Autodesk Fusion 360 part; units mm, degrees
note: some values were not read from the file. Set by a fixed rule: which face or edge a step refers to.
(part 3 of 4)
  circle A0 centre (-1.215, 0) radius 21.6
  circle A1 centre (-36.643, 0) radius 6.215
  circle A2 centre (-18.929, -30.6815) radius 6.215
  circle A3 centre (16.499, -30.6815) radius 6.215
  circle A4 centre (34.213, 0) radius 6.215
  circle A5 centre (16.499, 30.6815) radius 6.215
  circle A6 centre (-18.929, 30.6815) radius 6.215
  circle A7 centre (54, 0) radius 2
  circle A8 centre (53.3352, 8.4475) radius 2
  circle A9 centre (51.3571, 16.6869) radius 2
  circle A10 centre (48.1144, 24.5155) radius 2
  circle A11 centre (43.6869, 31.7404) radius 2
  circle A12 centre (38.1838, 38.1838) radius 2
  circle A13 centre (31.7404, 43.6869) radius 2
  circle A14 centre (24.5155, 48.1144) radius 2
  circle A15 centre (16.6869, 51.3571) radius 2
  circle A16 centre (8.4475, 53.3352) radius 2
  circle A17 centre (0, 54) radius 2
  circle A18 centre (-8.4475, 53.3352) radius 2
  circle A19 centre (-16.6869, 51.3571) radius 2
  circle A20 centre (-24.5155, 48.1144) radius 2
  circle A21 centre (-31.7404, 43.6869) radius 2
  circle A22 centre (-38.1838, 38.1838) radius 2
  circle A23 centre (-43.6869, 31.7404) radius 2
  circle A24 centre (-48.1144, 24.5155) radius 2
  circle A25 centre (-51.3571, 16.6869) radius 2
  circle A26 centre (-53.3352, 8.4475) radius 2
  circle A27 centre (-54, 0) radius 2
  circle A28 centre (-53.3352, -8.4475) radius 2
  circle A29 centre (-51.3571, -16.6869) radius 2
  circle A30 centre (-48.1144, -24.5155) radius 2
  circle A31 centre (-43.6869, -31.7404) radius 2
  circle A32 centre (-38.1838, -38.1838) radius 2
  circle A33 centre (-31.7404, -43.6869) radius 2
  circle A34 centre (-24.5155, -48.1144) radius 2
  circle A35 centre (-16.6869, -51.3571) radius 2
  circle A36 centre (-8.4475, -53.3352) radius 2
  circle A37 centre (0, -54) radius 2
  circle A38 centre (8.4475, -53.3352) radius 2
  circle A39 centre (16.6869, -51.3571) radius 2
  circle A40 centre (24.5155, -48.1144) radius 2
  circle A41 centre (31.7404, -43.6869) radius 2
  circle A42 centre (38.1838, -38.1838) radius 2
  circle A43 centre (43.6869, -31.7404) radius 2
  circle A44 centre (48.1144, -24.5155) radius 2
  circle A45 centre (51.3571, -16.6869) radius 2
  circle A46 centre (53.3352, -8.4475) radius 2
  circle A47 centre (-35.428, 0) radius 5
  circle A48 centre (-17.714, -30.6815) radius 5
  circle A49 centre (17.714, -30.6815) radius 5
  circle A50 centre (35.428, 0) radius 5
  circle A51 centre (17.714, 30.6815) radius 5
  circle A52 centre (-17.714, 30.6815) radius 5
  dimension "d277" = 35.428
  measures "d277" distance of origin A50.centre
sketch "outer teeth" plane through (0, 0, 0) normal (0, 0, 1) x (1, 0, 0) in component "ACG - Trapezoidal Profiles"
  line L0 (50.4, 0.75) -> (50.4, 0)
  circle A0 centre (0, 0) radius 55
  line L1 (54.9231, 2.9074) -> (50.4, 0.75)
  line L2 (0, 0) -> (55, 0) construction
  circle A1 centre (0, 0) radius 60
  line L3 (50.4, -0.75) -> (54.9231, -2.9074)
  line L4 (50.4, 0) -> (50.4, -0.75)
  dimension "d253" = 110
  dimension "d254" = 1.5
  dimension "d255" = 25.5
  dimension "d256" = 4.6
  dimension "d257" = 25.5
  dimension "d258" = 120
  constraint coincident A0.centre L2.start
  constraint coincident L2.end A0
  constraint horizontal L2
  constraint coincident L1.start A0
  constraint coincident L0.end L2
  constraint coincident L3.end A0
  constraint vertical L0
  constraint vertical L4
  constraint equal L0 L4
  measures "d253" diameter of A0
  measures "d254" distance of L3.start L0.start
  measures "d255" angle of L1 L2
  measures "d256" distance of L2.end L0
  measures "d257" angle of L2 L3
  measures "d258" diameter of A1
sketch "inner teeth" plane through (0, 0, 0) normal (0, 0, 1) x (1, 0, 0) in component "ACG - Trapezoidal Profiles"
  line L0 (2.7, 0) -> (50.046, 3.8222) construction
  line L1 (54.6914, 3.4447) -> (50.18, 1.3778)
  line L2 (2.7, 0) -> (50.2, 0) construction
  circle A0 centre (2.7, 0) radius 47.5
  line L3 (54.5707, 4.9399) -> (54.6914, 3.4447)
  line L4 (49.7862, 6.2564) -> (54.5707, 4.9399)
  point P0 (54.6311, 4.1923)
  dimension "d246" = 95
  dimension "d247" = 1.5
  dimension "d248" = 20
  dimension "d249" = 20
  dimension "d250" = 4.6
  dimension "d251" = 2.7
  dimension "d252" = 4.615
  constraint coincident L0.end A0
  constraint coincident L4.start A0
  constraint coincident L1.end A0
  constraint midpoint P0 L3
  constraint coincident L0.start L2.start
  constraint horizontal L0.start origin
  constraint coincident P0 L0
  constraint perpendicular L0 L3
  constraint coincident L2.end A0
  constraint horizontal L2
  measures "d246" diameter of A0
  measures "d247" distance of L1.start L3.start
  measures "d248" angle of L0 L4
  measures "d249" angle of L0 L1
  measures "d250" distance of L0.end L3
  measures "d251" distance of L0.start origin
  measures "d252" angle of L0 L2
sketch "Pins & Casing" plane through (0, 0, 0) normal (0, 0, 1) x (1, 0, 0) in component "Casing"
  circle A0 centre (-54, 0) radius 2
  circle A1 centre (0, 0) radius 55
  circle A2 centre (0, 0) radius 60
  line L0 (-35, -71) -> (-38.501, -76)
  line L1 (-60, -76) -> (-46.499, -76)
  line L2 (-60, -62) -> (-25, -42)
  circle A3 centre (0, 0) radius 15
  line L3 (-50, -71) -> (-35, -71)
  line L4 (-46.499, -76) -> (-50, -71)
  line L5 (50, -71) -> (46.499, -76)
  line L6 (-60, -80) -> (60, -80)
  line L7 (-60, -62) -> (60, -62)
  circle A4 centre (0, 0) radius 10
  line L8 (35, -71) -> (50, -71)
  line L9 (-38.501, -76) -> (38.501, -76)
  line L10 (46.499, -76) -> (60, -76)
  line L11 (25, -42) -> (60, -62)
  line L12 (-14.622, 3.3464) -> (-25, -42)
  line L13 (14.622, 3.3464) -> (25, -42)
  line L14 (38.501, -76) -> (35, -71)
  line L15 (-60, 0) -> (-60, -80)
  line L16 (60, -80) -> (60, 0)
  line L17 (54.9231, 2.9074) -> (50.4, 0.75)
  line L18 (50.4, 0.75) -> (50.4, 0)
  line L19 (50.4, 0) -> (50.4, -0.75)
  line L20 (50.4, -0.75) -> (54.9231, -2.9074)
  dimension "d9" = 110
  dimension "d10" = 120
  dimension "d33" = 80
  dimension "d34" = 30
  dimension "d35" = 20
  dimension "d36" = 55
  dimension "d37" = 55
  dimension "d38" = 55
  dimension "d39" = 55
  dimension "d40" = 4
  dimension "d41" = 5
  dimension "d42" = 10
  dimension "d43" = 15
  dimension "d44" = 18
  dimension "d45" = 20
  dimension "d50" = 25
  constraint coincident A1.centre A2.centre
  constraint perpendicular L6 L15
  constraint vertical L16
  constraint horizontal L6
  constraint coincident L2.start L15
  constraint coincident L7.end L16
  constraint coincident L13.start A3
  constraint coincident L12.start A3
  constraint tangent A3 L13
  constraint tangent A3 L12
  constraint coincident L1.start L15
  constraint perpendicular L1 L15
  constraint coincident L10.end L16
  constraint perpendicular L10 L16
  constraint horizontal L9
  constraint horizontal L3
  constraint horizontal L8
  constraint collinear L1 L9
  constraint collinear L9 L10
  constraint collinear L3 L8
  constraint equal L3 L8
  constraint equal L1 L10
  constraint horizontal L2.start L7.end
  constraint horizontal L2.end L11.start
  constraint equal L2 L11
  constraint coincident A2 L16.end
  constraint coincident A2 L15.start
  constraint tangent A2 L15
  constraint tangent A2 L16
  measures "d9" diameter of A1
  measures "d10" diameter of A2
  measures "d33" distance of A1.centre L6
  measures "d34" diameter of A3
  measures "d35" diameter of A4
  measures "d36" angle of L1 L4
  measures "d37" angle of L0 L9
  measures "d38" angle of L9 L14
  measures "d39" angle of L5 L10
  measures "d40" distance of L1 L6
  measures "d41" distance of L1 L3
  measures "d42" distance of L3.start L15
  measures "d43" distance of L3.start L0.start
  measures "d44" distance of L2.start L6
  measures "d45" vertical distance of L2.start L2.end
  measures "d50" horizontal distance of L2.end A1.centre
extrude "Extrude1" add sketch "Pins & Casing" against normal blind 5 contours A0 A1 | A0 A1 A2 L2 L11 | A1 L2 A3 L11 L12 L13 | A1 A2 L2 L11 | A2 L2 L15 | A2 L2 L7 L11 | A2 L11 L16 | L0 L1 L3 L4 L5 L7 L8 L9 L10 L14 L15 L16 | A3 | L0 L1 L3 L4 L5 L6 L8 L9 L10 L14 L15 L16 picked at (-55.3296, 0.0472) makes body 1 in component "Casing"
extrude "Extrude2" add sketch "Pins & Casing" against normal up to surface (5 mm away) contours A1 L17 L18 L19 L20 bodies 1 in component "Casing"
pattern_circular "C-Pattern1" count 40 over 360 about axis through (0, 0, 1.75) along (0, 0, 1) of "Extrude2" in component "Casing"
extrude "Extrude3" add sketch "Pins & Casing" along normal blind 24 contours A0 A1 | A0 A1 A2 L2 L11 | A1 A2 L2 L11 | A2 L2 L15 | A2 L2 L7 L11 | A2 L11 L16 | L0 L1 L3 L4 L5 L7 L8 L9 L10 L14 L15 L16 | L0 L1 L3 L4 L5 L6 L8 L9 L10 L14 L15 L16 picked at (-55.3296, 0.0472) bodies 1 in component "Casing"
extrude "Extrude7" add sketch "Pins & Casing" along normal up to surface (24 mm away) contours A1 L17 L18 L19 L20 bodies 1 in component "Casing"
fillet "Fillet3" radius 1 2 edges at (50.4, 0.75, 9.5) (50.4, -0.75, 9.5) on bodies 1 in component "Casing"
fillet "Fillet4" radius 1 2 edges at (54.9231, 2.9074, 9.5) (54.9231, -2.9074, 9.5) on bodies 1 in component "Casing"
pattern_circular "C-Pattern2" count 40 over 360 about axis through (0, 0, 1.75) along (0, 0, 1) of "Extrude7", "Fillet3", "Fillet4" in component "Casing"
extrude "Extrude8" add sketch "Pins & Casing" along normal blind 25 from surface at 24 contours L0 L1 L3 L4 L5 L7 L8 L9 L10 L14 L15 L16 | L0 L1 L3 L4 L5 L6 L8 L9 L10 L14 L15 L16 bodies 1 in component "Casing"
extrude "Extrude4" cut sketch "Pins & Casing" against normal blind 30 from surface at 49 contours L0 L1 L3 L4 L5 L6 L8 L9 L10 L14 L15 L16 bodies 1 in component "Casing"
extrude "Extrude5" add sketch "Pins & Casing" along normal up to surface (30 mm away) from surface at 19 separate body contours L0 L1 L3 L4 L5 L6 L8 L9 L10 L14 L15 L16 makes body 2 in component "Casing"
extrude "Extrude6" add sketch "Pins & Casing" along normal blind 5 from surface at 49 contours A1 L2 A3 L11 L12 L13 | A1 A2 L2 L11 | A2 L2 L7 L11 | L0 L1 L3 L4 L5 L7 L8 L9 L10 L14 L15 L16 | A3 | L0 L1 L3 L4 L5 L6 L8 L9 L10 L14 L15 L16 bodies 2 in component "Casing"
fillet "Fillet1" radius 0.6 4 edges at (50, -71, 34) (35, -71, 34) (-35, -71, 34) (-50, -71, 34) on bodies 2 in component "Casing"
fillet "Fillet2" radius 0.6 4 edges at (-46.499, -76, 34) (-38.501, -76, 34) (38.501, -76, 34) (46.499, -76, 34) on bodies 1 in component "Casing"
chamfer "Chamfer1" distance 3 angle 45 16 edges at (-19.811, -19.3268, 54) (19.811, -19.3268, 54) (0, 15, 54) (-42.5, -52, 54) (42.5, -52, 54) (60, -71, 54) (-60, -71, 54) (0, 60, -5) (60, -40, -5) (-60, -40, -5) (0, 60, 24) (-60, -31, 24) (60, -31, 24) (19.811, -19.3268, -5) (-19.811, -19.3268, -5) (0, 15, -5) measured on face at (8.3333, -67.3333, 54) measured on face at (8.3333, -67.3333, 54) measured on face at (8.3333, -67.3333, 54) measured on face at (8.3333, -67.3333, 54) measured on face at (8.3333, -67.3333, 54) measured on face at (8.3333, -67.3333, 54) measured on face at (8.3333, -67.3333, 54) measured on face at (-9.8854, -68.2202, -5) measured on face at (-9.8854, -68.2202, -5) measured on face at (-9.8854, -68.2202, -5) measured on face at (1.1951, -59.6277, 24) measured on face at (1.1951, -59.6277, 24) measured on face at (1.1951, -59.6277, 24) measured on face at (-9.8854, -68.2202, -5) measured on face at (-9.8854, -68.2202, -5) measured on face at (-9.8854, -68.2202, -5) on bodies 1 2 in component "Casing"
sketch "Sketch1" plane through (0, 0, 0) normal (0, 0, 1) x (1, 0, 0) in component "Shaft"
  circle A0 centre (0, 0) radius 10
  line L0 (3.35, 1.9341) -> (0, 3.8682)
  line L1 (0, 3.8682) -> (-3.35, 1.9341)
  line L2 (-3.35, 1.9341) -> (-3.35, -1.9341)
  line L3 (-3.35, -1.9341) -> (0, -3.8682)
  line L4 (0, -3.8682) -> (3.35, -1.9341)
  line L5 (3.35, -1.9341) -> (3.35, 1.9341)
  circle A1 centre (2.7, 0) radius 21.6
  circle A2 centre (0, 0) radius 12
  circle A3 centre (0, 7.4) radius 1.5
  circle A4 centre (-2.7, 0) radius 21.6
  dimension "d61" = 20
  dimension "d62" = 3.35
  dimension "d65" = 43.2
  dimension "d66" = 2.7
  dimension "d68" = 24
  dimension "d69" = 3
  dimension "d70" = 7.4
  dimension "d279" = 43.2
  dimension "d280" = 2.7
  constraint coincident A0.centre A2.centre
  constraint vertical L5
  constraint horizontal A0.centre A1.centre
  constraint vertical A0.centre A3.centre
  constraint horizontal A0.centre A4.centre
  measures "d61" diameter of A0
  measures "d62" distance of A0.centre L5
  measures "d65" diameter of A1
  measures "d66" distance of A0.centre A1.centre
  measures "d68" diameter of A2
  measures "d69" diameter of A3
  measures "d70" distance of A0.centre A3.centre
  measures "d279" diameter of A4
  measures "d280" distance of A0.centre A4.centre
extrude "Extrude1'" add sketch "Sketch1" along normal blind 10 from surface at 4 separate body contours A0 | L0 L1 L2 L3 L4 L5 | A1 A4 | A1 A4 | A2 | A3 picked at (1.3185, 18.0717) picked at (-22.4609, 0) makes body 3 in component "Shaft"
extrude "Extrude2'" add sketch "Sketch1" along normal blind 10 from surface at 14 contours A0 | L0 L1 L2 L3 L4 L5 | A1 A4 | A1 A4 | A2 | A3 picked at (20.0404, 5.0981) picked at (1.3185, 18.0717) bodies 3 in component "Shaft"
extrude "Extrude3'" add sketch "Sketch1" along normal blind 50 from surface at 24 contours A0 | L0 L1 L2 L3 L4 L5 | A3 bodies 3 in component "Shaft"
extrude "Extrude4'" cut sketch "Sketch1" along normal blind 15 from surface at 4 contours A0 | L0 L1 L2 L3 L4 L5 | A3 bodies 3 in component "Shaft"
chamfer "Chamfer1'" distance 7 angle 55 1 edges at (-9.3233, -3.6162, 19) measured on face at (9.9503, -0.9957, 14) on bodies 3 in component "Shaft"
extrude "Extrude5'" add sketch "Sketch1" along normal blind 17 from surface at -5 separate body contours A0 | L0 L1 L2 L3 L4 L5 | A3 makes body 4 in component "Shaft"
chamfer "Chamfer2" distance 0.75 angle 45 1 edges at (-9.3233, -3.6162, 12) measured on face at (2.3712, -3.5556, 12) on bodies 4 in component "Shaft"
extrude "Extrude6'" cut sketch "Sketch1" against normal blind 30 from surface at 74 contours L0 L1 L2 L3 L4 L5 bodies 3 in component "Shaft"
extrude "Extrude7'" cut sketch "Sketch1" against normal blind 1 from surface at 74 contours A3 bodies 3 in component "Shaft"
move_body "Move1" bodies 3 to x (-1, 0, 0) y (0, -1, 0) z (0, 0, 1) at (0, 0, 0) in component "Shaft"
sketch "Sketch1 (2)" plane through (0, 0, 0) normal (0, 0, 1) x (1, 0, 0) in component "Cycloidal Discs"
  arc A0 (-51.8001, -0.0065) -> (-51.8028, 0.0333) centre (-52, 0) ccw
  circle A1 centre (2.7, 45) radius 1.5
  circle A2 centre (2.7, 0) radius 47.5
  line L0 (54.5707, 4.9399) -> (54.6914, 3.4447)
  line L1 (54.6914, 3.4447) -> (50.18, 1.3778)
  line L2 (49.7862, 6.2564) -> (54.5707, 4.9399)
  circle A3 centre (2.7, 0) radius 21.8
  line L3 (2.7, 0) -> (2.7, 47.5) construction
  circle A4 centre (38.128, 0) radius 7.7
  line L4 (2.7, 0) -> (50.046, 3.8222) construction
  line L5 (2.7, 0) -> (50.2, 0) construction
  dimension "d157" = 3
  dimension "d259" = 43.6
  dimension "d260" = 2.5
  dimension "d261" = 15.4
  dimension "d262" = 35.428
  constraint concentric A2 A3
  constraint coincident A2.centre A3.centre
  constraint coincident A2 L3.end
  constraint vertical L3
  constraint coincident A1.centre L3
  constraint coincident A2 L5.end
  constraint horizontal L5
  constraint coincident A4.centre L5
  measures "d157" diameter of A1
  measures "d259" diameter of A3
  measures "d260" distance of A1.centre L3.end
  measures "d261" diameter of A4
  measures "d262" distance of A2.centre A4.centre
extrude "Extrude1''" add sketch "Sketch1 (2)" along normal blind 10 from surface at 4 separate body contours A1 | A2 | A4 makes body 5 in component "Cycloidal Discs"
extrude "Extrude9" add sketch "Sketch1 (2)" along normal up to surface (10 mm away) from surface at 4 contours A2 L0 L1 L2 bodies 5 in component "Cycloidal Discs"
fillet "Fillet1'" radius 0.4 2 edges at (54.6914, 3.4447, 9) (54.5707, 4.9399, 9) on bodies 5 in component "Cycloidal Discs"
fillet "Fillet2'" radius 1.6 2 edges at (49.7862, 6.2564, 9) (50.18, 1.3778, 9) on bodies 5 in component "Cycloidal Discs"
pattern_circular "C-Pattern1'" count 39 over 360 about axis through (2.7, 0, 4) along (0, 0, 1) of "Extrude9", "Fillet1'", "Fillet2'" in component "Cycloidal Discs"
extrude "Extrude10" cut sketch "Sketch1 (2)" along normal up to surface (14 mm away) contours A4 bodies 5 in component "Cycloidal Discs"
pattern_circular "C-Pattern2'" count 6 over 360 about axis through (2.7, 0, 4) along (0, 0, 1) of "Extrude10" in component "Cycloidal Discs"
extrude "Extrude3''" cut sketch "Sketch1 (2)" against normal blind 1 from surface at 14 contours A1 bodies 5 in component "Cycloidal Discs"
copy_body "CopyPasteBodies1" bodies 5 makes body 6 in component "Cycloidal Discs"
move_body "Move3" bodies 6 to x (-1, 0, 0) y (0, -1, 0) z (0, 0, 1) at (5.4, 0, 0) in component "Cycloidal Discs"
move_body "Move4" bodies 6 to x (1, 0, 0) y (0, 1, 0) z (0, 0, 1) at (-5.4, 0, 0) in component "Cycloidal Discs"
move_body "Move5" bodies 6 to x (1, 0, 0) y (0, 1, 0) z (0, 0, 1) at (0, 0, 10) in component "Cycloidal Discs"
sketch "Sketch1 (3)" plane through (0, 0, 0) normal (0, 0, 1) x (1, 0, 0) in component "Output"
  circle A0 centre (35.428, 0) radius 5
  circle A1 centre (0, 0) radius 40.428
  circle A2 centre (0, 0) radius 10
  circle A3 centre (0, 0) radius 15
  circle A4 centre (38, 0) radius 1.5
  line L0 (0, 0) -> (35.428, 0) construction
  circle A5 centre (35.428, 0) radius 2.5
  line L1 (14.1421, 5) -> (35.428, 5)
  line L2 (35.428, -5) -> (14.1421, -5)
  dimension "d110" = 20
  dimension "d123" = 30
  dimension "d165" = 3
  dimension "d166" = 38
  dimension "d204" = 5
  constraint coincident A1.centre A2.centre
  constraint concentric A1 A2
  constraint coincident A0.centre L0.end
  constraint concentric A0 A5
  constraint tangent A0 A1
  constraint coincident A3 L1.start
  constraint coincident A0 L1.end
  constraint coincident A0 L2.start
  constraint coincident A3 L2.end
  constraint horizontal L2
  constraint horizontal L1
  constraint tangent A0 L1
  constraint tangent A0 L2
  constraint coincident A4.centre L0
  measures "d110" diameter of A2
  measures "d123" diameter of A3
  measures "d165" diameter of A4
  measures "d166" distance of A1.centre A4.centre
  measures "d204" diameter of A5
extrude "Extrude1'''" add sketch "Sketch1 (3)" along normal up to surface (4 mm away) separate body contours A3 makes body 7 in component "Output"
extrude "Extrude8'" add sketch "Sketch1 (3)" along normal up to surface (4 mm away) contours A0 | A0 A3 L1 L2 | A4 A5 | A4 A5 | A4 A5 bodies 7 in component "Output"
extrude "Extrude2''" add sketch "Sketch1 (3)" along normal up to surface (24 mm away) contours A0 | A4 A5 | A4 A5 | A4 A5 bodies 7 in component "Output"
extrude "Extrude9'" add sketch "Sketch1 (3)" along normal blind 7 from surface at 24 contours A4 A5 | A4 A5 picked at (37.4543, 0.2317) picked at (34.1293, 0.1601) bodies 7 in component "Output"
chamfer "Chamfer4" distance 0.8 angle 45 1 edges at (33.0972, -0.904, 31) measured on face at (34.7636, 0.7403, 31) on bodies 7 in component "Output"
fillet "Fillet4'" radius 4 2 edges at (14.1421, 5, 2) (14.1421, -5, 2) on bodies 7 in component "Output"
pattern_circular "C-Pattern2''" count 6 over 360 about axis through (0, 0, 1.75) along (0, 0, 1) of "Extrude8'", "Extrude2''", "Extrude9'", "Chamfer4", "Fillet4'" in component "Output"
extrude "Extrude3'''" add sketch "Sketch1 (3)" along normal blind 10 from surface at 24 separate body contours A3 makes body 8 in component "Output"